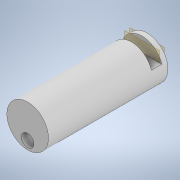
# Autodesk Inventor part: lamp2
Saved by Autodesk Inventor 2020 (Build 240168000, 168)
## iProperties
Created: 2022-10-15
Part Number: lamp2
Material: Типовые
Document SubType Name: Modeling
Designer: zigma
Density: 1 g/cm^3
Appearance: По умолчанию
Author: zigma
Autodesk Inventor part; units mm, degrees
ref_plane "YZ Plane" through (0, 0, 0) normal (1, 0, 0) x (0, 1, 0)
ref_plane "XZ Plane" through (0, 0, 0) normal (0, 1, 0) x (-1, 0, 0)
ref_plane "XY Plane" through (0, 0, 0) normal (0, 0, 1) x (1, 0, 0)
sketch "Эскиз1" plane through (0, 0, 0) normal (0, 0, 1) x (1, 0, 0)
  arc A0 (47.2167, -13.0271) -> (19.1654, -13.0271) centre (33.1911, 1.2306) ccw
  line L0 (26.6911, 1.9729) -> (39.6911, 1.9729)
  line L1 (39.6911, 1.9729) -> (42.6385, -9.0271)
  line L2 (33.1911, 1.9729) -> (33.1911, -13.0271) construction
  line L3 (26.6911, 1.9729) -> (23.7436, -9.0271)
  line L4 (22.6718, -13.0271) -> (22.6718, -11.0271)
  line L5 (22.6718, -11.0271) -> (20.6718, -11.0271)
  line L6 (20.6718, -11.0271) -> (20.6718, -9.0271)
  line L7 (20.6718, -9.0271) -> (23.7436, -9.0271)
  line L8 (43.7103, -13.0271) -> (43.7103, -11.0271)
  line L9 (43.7103, -11.0271) -> (45.7103, -11.0271)
  line L10 (45.7103, -11.0271) -> (45.7103, -9.0271)
  line L11 (45.7103, -9.0271) -> (42.6385, -9.0271)
  line L12 (19.1654, -13.0271) -> (22.6718, -13.0271)
  line L13 (43.7103, -13.0271) -> (47.2167, -13.0271)
  point P0 (19.1654, -13.0271)
  dimension "d3" = 13
  dimension "d4" = 105
  dimension "d5" = 15
  dimension "d6" = 40
  dimension "d44" = 2
  dimension "d45" = 2
  dimension "d46" = 2
  dimension "d47" = 3.5064
  constraints: 28 end point, 5 symmetric about line, 3 horizontal, 3 perpendicular, 2 point on circle, 2 vertical, 1 centre point, 1 midpoint, 1 other
  measures "d3" distance of L0.start L0.end
  measures "d4" angle of L0 L1
  measures "d5" distance from line of A0.end L0
  measures "d6" diameter of A0
  measures "d44" distance of L4.start L4.end
  measures "d45" distance of L4.end L5.end
  measures "d46" distance of L5.end L6.end
  measures "d47" distance of L4.start A0.end
extrude "Выдавливание1" add sketch "Эскиз1" along normal blind 200
ref_plane "РабПлоскость2" through (0, 0, 105) normal (0, 0, 1) x (1, 0, 0)
ref_plane "РабПлоскость1" through (0, 0, 100) normal (0, 0, 1) x (1, 0, 0)
sketch "Эскиз3" plane through (0, 0, 200) normal (0, 0, 1) x (1, 0, 0)
  arc A0 (47.2167, -13.0271) -> (19.1654, -13.0271) centre (33.1911, 1.2306) ccw projected
  circle A1 centre (33.1911, 1.2306) radius 20
  point P0 (0, 0)
  point P1 (19.1654, -13.0271)
  constraints: 1 coincident, 3 other
extrude "Выдавливание3" add sketch "Эскиз3" along normal blind 15
sketch "Эскиз5" plane through (33.1911, 1.2306, 215) normal (0, 0, 1) x (1, 0, 0)
  circle A0 centre (0, -12) radius 6
  circle A1 centre (0, 0) radius 20 construction
  circle A2 centre (0, 0) radius 18 construction
  circle A3 centre (0, 0) radius 20 construction
  line L0 (0, -20) -> (0, 0)
  point P0 (-33.1911, -1.2306)
  dimension "d38" = 12
  dimension "d39" = 2
  constraints: 3 centre point, 2 end point, 1 coincident, 1 point on line, 1 tangent, 1 vertical, 1 vertical alignment, 2 other
  measures "d38" diameter of A0
  measures "d39" radial gap between concentric circles of A1 A2
extrude "Выдавливание5" cut sketch "Эскиз5" against normal blind 15
sketch "Эскиз13" plane through (0, 0, 105) normal (0, 0, 1) x (1, 0, 0)
  circle A0 centre (33.1911, 1.2306) radius 20 projected
  circle A1 centre (33.1911, 1.2306) radius 20
  line L0 (14.1123, 7.2306) -> (52.2699, 7.2306)
  point P0 (0, 0)
  dimension "d79" = 6
  constraints: 2 end point, 2 point on circle, 1 centre point, 1 coincident, 1 concentric, 1 horizontal
  measures "d79" distance from line of L0 A1.centre
extrude "Выдавливание12" cut sketch "Эскиз13" along normal blind 10 contours L0 A0 picked at (30.9346, 14.3004)
sketch "Эскиз14" plane through (0, 0, 0) normal (0, 0, -1) x (-1, 0, 0)
  arc A0 (-14.1123, 7.2306) -> (-52.2699, 7.2306) centre (-33.1911, 1.2306) ccw projected
  circle A1 centre (-33.1911, 1.2306) radius 20
  point P0 (0, 0)
  point P1 (-52.2699, 7.2306)
  constraints: 1 centre point, 1 coincident, 1 concentric
extrude "Выдавливание13" cut sketch "Эскиз14" against normal up to surface (100 mm away)
sketch "Эскиз15" plane through (33.1911, 1.2306, 100) normal (0, 0, -1) x (-1, 0, 0)
  line L0 (-5, 11) -> (5, 11)
  line L1 (5, 11) -> (5, 6)
  line L2 (5, 6) -> (-5, 6)
  line L3 (-5, 6) -> (-5, 11)
  arc A0 (19.0788, 6) -> (-19.0788, 6) centre (0, 0) ccw projected
  line L4 (0, 0) -> (0, 22.3404)
  point P0 (33.1911, -1.2306)
  point P1 (0, 11)
  dimension "d84" = 10
  dimension "d85" = 5
  dimension "d86" = 6
  constraints: 10 end point, 2 parallel, 1 horizontal, 1 midpoint, 1 perpendicular, 1 point on line, 1 vertical
  measures "d84" distance of L1.end L2.end
  measures "d85" distance of L0.end L1.end
  measures "d86" distance from line of L4.start L2
extrude "Выдавливание14" add sketch "Эскиз15" along normal blind 5
